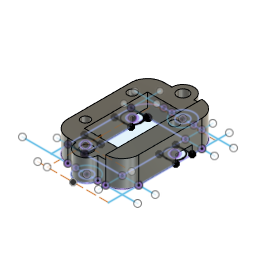
volume-holder (Autodesk Fusion 360 design; units mm, degrees)
Autodesk Fusion 360 part; units mm, degrees
note: some values were not read from the file. Set by a fixed rule: which sketch regions a step uses.
sketch "Skizze1" plane through (0, 0, 0) normal (0, 0, 1) x (1, 0, 0)
  circle A0 centre (-13, 14) radius 1.6
  circle A1 centre (-13, -3) radius 1.6
  line L0 (-10.4, 17) -> (-10.4, -6)
  line L1 (-11.4, 14) -> (-10.4, 14) construction
  line L2 (-19, 17) -> (14, 17)
  line L3 (-20.3748, -6) -> (15.4156, -6)
  line L4 (-16.4, 27.5706) -> (-16.4, -12)
  line L5 (-11.401, -2.9445) -> (3.799, -2.9445) construction
  line L6 (3.4, -14.6443) -> (3.4, 27)
  line L7 (9.4, 27) -> (9.4, -17)
  line L8 (-21, 23) -> (15, 23)
  line L9 (15, -12) -> (-27, -12)
  circle A2 centre (6, 10.5) radius 1.6
  line L10 (4.4, 10.5) -> (3.4, 10.5) construction
  line L11 (-13, -3) -> (-13, 3) construction
  line L12 (-13, 3) -> (-13, -17) construction
  line L13 (9.4, -17) -> (-16.4, -17) construction
  line L14 (-13, 3) -> (-13, 23) construction
  line L15 (-16.4, 22.0964) -> (9.4, 22.0964) construction
  line L16 (-3.5, 22.0964) -> (-3.5, 23) construction
  circle A3 centre (-3.5, 23) radius 2.05
  circle A4 centre (-3.5, 23) radius 4
  circle A5 centre (-3.5, -12) radius 2.05
  circle A6 centre (-3.5, -12) radius 4
  point P0 (-3.5, -17)
  point P1 (-3.5, 22.0964)
  dimension "d1" = 3.2
  dimension "d2" = 3.2
  dimension "d3" = 17
  dimension "d4" = 1
  dimension "d5" = 3
  dimension "d6" = 3
  dimension "d7" = 6
  dimension "d8" = 15.2
  dimension "d9" = 6
  dimension "d10" = 6
  dimension "d11" = 6
  dimension "d12" = 3.2
  dimension "d13" = 3.5
  dimension "d16" = 2.6
  dimension "d21" = 6
  dimension "d22" = 20
  dimension "d24" = 25.8
  dimension "d27" = 20
  dimension "d28" = 4.1
  dimension "d29" = 8
  dimension "d40" = 4.1
  dimension "d41" = 8
  constraint vertical A0.centre A1.centre
  constraint vertical L0
  constraint coincident A0 L1.start
  constraint coincident L0 L1.end
  constraint perpendicular L0 L1
  constraint horizontal L2
  constraint perpendicular L0 L3
  constraint perpendicular L3 L4
  constraint coincident A1 L5.start
  constraint perpendicular L0 L5
  constraint perpendicular L2 L6
  constraint vertical L7
  constraint horizontal L8
  constraint horizontal L9
  constraint coincident L4.end L9
  constraint coincident A2 L10.start
  constraint coincident L6 L10.end
  constraint perpendicular L6 L10
  constraint coincident L0.start L2
  constraint coincident L0.end L3
  constraint coincident A1.centre L11.start
  constraint parallel L0 L11
  constraint perpendicular L9 L12
  constraint perpendicular L4 L13
  constraint midpoint L13 P0
  constraint horizontal L12.end P0
  constraint perpendicular L8 L14
  constraint coincident L4 L15.start
  constraint coincident L7 L15.end
  constraint perpendicular L7 L15
  constraint midpoint L15 P1
  constraint coincident P1 L16.start
  constraint coincident L8 L16.end
  constraint perpendicular L8 L16
  constraint coincident L16.end A3.centre
  constraint concentric A3 A4
  constraint coincident L9 A5.centre
  constraint concentric A5 A6
  measures "d1" diameter of A0
  measures "d2" diameter of A1
  measures "d3" distance of A0.centre A1.centre
  measures "d4" distance of L1.start L1.end
  measures "d5" distance of A0.centre L2
  measures "d6" distance of A1.centre L3
  measures "d7" distance of L0 L4
  measures "d8" distance of L5.start L5.end
  measures "d9" distance of L6 L7
  measures "d10" distance of L2 L8
  measures "d11" distance of L3 L9
  measures "d12" diameter of A2
  measures "d13" vertical distance of A0.centre A2.centre
  measures "d16" distance of L6 A2.centre
  measures "d21" distance of A1.centre L11.end
  measures "d22" distance of L11.end L12.end
  measures "d24" distance of L7.end L13.end
  measures "d27" distance of L11.end L14.end
  measures "d28" diameter of A3
  measures "d29" diameter of A4
  measures "d40" diameter of A5
  measures "d41" diameter of A6
extrude "Extrusion1" add sketch "Skizze1" along normal blind 8 contours L0 L2 L3 L4 | L2 L4 L6 L8 A4 | L3 L4 L6 L9 A6 | L2 L6 L7 L8 | L2 L3 L6 L7 | L3 L6 L7 L9 | L8 A3 A4 | L9 A5 A6 | L8 A3 | L9 A5 picked at (-0.1725, 22.6994) picked at (-6.7682, -11.3064) picked at (-3.4489, 22.3186) picked at (-2.9991, -11.3315)
extrude "Extrusion2" add sketch "Skizze1" along normal blind 9.6 contours L2 L6 L7 L8 | L2 L3 L6 L7 | L3 L6 L7 L9
extrude "Extrusion3" add sketch "Skizze1" along normal blind 8 contours L8 A3 A4 | L9 A5 A6 picked at (-6.8275, 23.3006) picked at (-6.8351, -12.1987)
extrude "Extrusion7" cut sketch "Skizze1" along normal blind 8 contours L8 A3 | L9 A5 picked at (-3.4489, 22.3186) picked at (-2.9991, -11.3315)
fillet "Abrundung2" radius 6 4 edges at (-16.4, -12, 4) (-16.4, 23, 4) (9.4, 23, 4.8) (9.4, -12, 4.8)
sketch "Skizze2" plane through (0, 0, 0) normal (0, 0, -1) x (1, 0, 0)
  circle A0 centre (-13, -14) radius 1.6
  circle A1 centre (-13, 3) radius 1.6
  line L0 (3.4, 6) -> (3.4, -17)
  line L1 (3.4, -17) -> (-10.4, -17)
  line L2 (-10.4, -17) -> (-10.4, 6)
  line L3 (-10.4, 6) -> (3.4, 6)
  circle A2 centre (6, -10.5) radius 1.6
  arc A3 (9.4, 6) -> (3.4, 12) centre (3.4, 6) ccw
  line L4 (3.4, 12) -> (0.5, 12)
  arc A4 (0.5, 12) -> (-7.5, 12) centre (-3.5, 12) ccw
  line L5 (-7.5, 12) -> (-10.4, 12)
  arc A5 (-10.4, 12) -> (-16.4, 6) centre (-10.4, 6) ccw
  line L6 (-16.4, 6) -> (-16.4, -17)
  arc A6 (-16.4, -17) -> (-10.4, -23) centre (-10.4, -17) ccw
  line L7 (-10.4, -23) -> (-7.5, -23)
  arc A7 (-7.5, -23) -> (0.5, -23) centre (-3.5, -23) ccw
  line L8 (0.5, -23) -> (3.4, -23)
  arc A8 (3.4, -23) -> (9.4, -17) centre (3.4, -17) ccw
  line L9 (9.4, -17) -> (9.4, 6)
  circle A9 centre (-3.5, 12) radius 2.05
  circle A10 centre (-3.5, -23) radius 2.05
  circle A11 centre (-13, 3) radius 3
  circle A12 centre (-13, -14) radius 3
  circle A13 centre (6, -10.5) radius 3
  line L10 (-10, 3) -> (-10, 6)
  line L11 (-10, -14) -> (-10, -17)
  line L12 (-13, 6) -> (-10.4, 6)
  line L13 (-13, 0) -> (-10.4, 0)
  line L14 (6, -7.5) -> (3.4, -7.5)
  line L15 (-13, -11) -> (-10.4, -11)
  line L16 (-13, -17) -> (-10.4, -17)
  line L17 (6, -13.5) -> (3.4, -13.5)
  line L18 (-13, 6) -> (-16.4, 6)
  line L19 (-13, 0) -> (-16.4, 0)
  line L20 (6, -7.5) -> (9.4, -7.5)
  line L21 (6, -13.5) -> (9.4, -13.5)
  line L22 (-13, -17) -> (-16.4, -17)
  line L23 (-13, -11) -> (-16.4, -11)
  dimension "d46" = 1.4
  dimension "d47" = 1.4
  dimension "d48" = 1.4
  constraint coincident A11 L10.start
  constraint coincident L3 L10.end
  constraint tangent A11 L10
  constraint perpendicular L3 L10
  constraint coincident A12 L11.start
  constraint coincident L1 L11.end
  constraint tangent A12 L11
  constraint perpendicular L1 L11
  constraint coincident A11 L12.start
  constraint coincident L2 L3.start
  constraint tangent A11 L12
  constraint perpendicular L2 L12
  constraint coincident A11 L13.start
  constraint coincident L2 L13.end
  constraint tangent A11 L13
  constraint perpendicular L2 L13
  constraint coincident A13 L14.start
  constraint coincident L0 L14.end
  constraint tangent A13 L14
  constraint perpendicular L0 L14
  constraint coincident A12 L15.start
  constraint coincident L2 L15.end
  constraint tangent A12 L15
  constraint perpendicular L2 L15
  constraint coincident A12 L16.start
  constraint coincident L1.end L2.start
  constraint tangent A12 L16
  constraint coincident A13 L17.start
  constraint coincident L0 L17.end
  constraint tangent A13 L17
  constraint perpendicular L0 L17
  constraint coincident A5.end L6.start
  constraint coincident L6 L19.end
  constraint tangent A11 L19
  constraint coincident L9 L20.end
  constraint tangent A13 L20
  constraint coincident L9 L21.end
  constraint tangent A13 L21
  constraint coincident L6.end A6.start
  constraint coincident L6 L23.end
  constraint tangent A12 L23
extrude "Extrusion8" cut sketch "Skizze2" against normal blind 3 contours L0 A13 L14 | L0 A13 | L9 A13 L20 L21 | L2 A11 L12 | L0 A13 L17 | L2 A11 | L6 A11 L18 L19 | L2 A11 L13 | L2 A12 L15 | L6 A12 L22 L23 | L2 A12 | L2 A12 L16 picked at (3.7333, -10.5) picked at (-10.7333, 3) picked at (-10.7333, -14)
